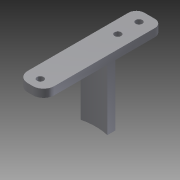
# Autodesk Inventor part: arm
Saved by Autodesk Inventor 2012 (Build 160160000, 160)
## iProperties
Created: 2014-03-21
Part Number: arm
Material: Default
Document SubType Name: Modeling
Designer: joe_000
Density: 1 g/cm^3
Author: joe_000
Autodesk Inventor part; units mm, degrees
ref_plane "YZ Plane" through (0, 0, 0) normal (1, 0, 0) x (0, 1, 0)
ref_plane "XZ Plane" through (0, 0, 0) normal (0, 1, 0) x (-1, 0, 0)
ref_plane "XY Plane" through (0, 0, 0) normal (0, 0, 1) x (1, 0, 0)
sketch "Sketch1" plane through (0, 0, 0) normal (0, 0, 1) x (1, 0, 0)
  line L0 (4, 0) -> (6, 0)
  line L1 (10, 4) -> (10, 42)
  line L2 (7, 45) -> (3, 45)
  line L3 (0, 42) -> (0, 4)
  arc A0 (0, 4) -> (4, 0) centre (4, 4) ccw
  arc A1 (6, 0) -> (10, 4) centre (6, 4) ccw
  arc A2 (3, 45) -> (0, 42) centre (3, 42) ccw
  arc A3 (10, 42) -> (7, 45) centre (7, 42) ccw
  point P0 (0, 0)
  point P1 (10, 45)
  point P2 (10, 0)
  point P3 (0, 45)
  dimension "d0" = 10
  dimension "d1" = 45
  dimension "d21" = 4
  dimension "d26" = 3
  constraints: 8 end point, 8 point on circle, 8 point on line, 8 tangent, 4 centre point, 2 equal radius, 2 parallel, 1 horizontal, 1 perpendicular
  measures "d0" distance of point (0, 0) point (10, 0)
  measures "d1" distance of point (10, 0) point (10, 45)
  measures "d21" radius of A0
  measures "d26" radius of A2
extrude "Extrusion1" add sketch "Sketch1" along normal blind 3
sketch "Sketch2" plane through (0, 0, 3) normal (0, 0, 1) x (1, 0, 0)
  circle A0 centre (5, 3.75) radius 1.25
  line L0 (0, 4) -> (0, 42) projected
  line L1 (6, 0) -> (4, 0) projected
  line L2 (3, 45) -> (7, 45) projected
  circle A1 centre (5, 33) radius 1.25
  circle A2 centre (5, 41) radius 1.25
  point P0 (0, 40)
  point P1 (0, 0)
  point P2 (10, 0)
  dimension "d4" = 2.5
  dimension "d14" = 3.75
  dimension "d18" = 5
  dimension "d27" = 2.5
  dimension "d28" = 2.5
  dimension "d29" = 4
  dimension "d30" = 8
  constraints: 3 centre point
  measures "d4" diameter of A0
  measures "d14" distance from line of L1 A0.centre
  measures "d18" distance from line of L0 A0.centre
  measures "d27" diameter of A2
  measures "d28" diameter of A1
  measures "d29" distance from line of L2 A2.centre
  measures "d30" distance of A1.centre A2.centre
extrude "Extrusion4" cut sketch "Sketch2" against normal through all
sketch "Sketch3" plane through (0, 0, 0) normal (0, 0, -1) x (-1, 0, 0)
  circle A0 centre (-5, 3.75) radius 1.25 projected
  line L0 (-10, 4) -> (-10, 42) projected
  line L1 (0, 42) -> (0, 4) projected
  arc A1 (0, 24.0323) -> (-10, 24.0323) centre (-5, 3.75) ccw
  arc A2 (0, 27.1104) -> (-10, 27.1104) centre (-5, 3.75) ccw
  point P0 (-10, 40)
  point P1 (0, 40)
  point P2 (0, 0)
  dimension "d22" = 20.8895
  dimension "d23" = 3
  constraints: 4 point on circle, 4 point on line, 2 centre point, 2 coincident
  measures "d22" radius of A1
  measures "d23" radial gap between concentric circles of A2 A1
extrude "Extrusion5" add sketch "Sketch3" along normal blind 23 contours L0 A2 L1 A1
equation "\"d4\" = centerHoleDia"
equation "\"d22\" = setScrewRingRad"
equation "\"d23\" = wallThickness"
equation "\"d24\" = wallHeight + wallThickness"
equation "\"centerHoleDia\" = 2.5"
equation "\"setScrewRingRad\" = 20.889512"
equation "\"wallThickness\" = 3"
equation "\"wallHeight\" = 20"
body "Solid1"
